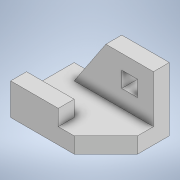
# Autodesk Inventor part: 零件12
Saved by Autodesk Inventor 2020 (Build 240168000, 168)
## iProperties
Created: 2020-09-19
Part Number: 零件12
Material: 一般
Document SubType Name: Modeling
Designer: User
Density: 1 g/cm^3
Appearance: 預設
Author: User
Autodesk Inventor part; units mm, degrees
ref_plane "YZ Plane" through (0, 0, 0) normal (1, 0, 0) x (0, 1, 0)
ref_plane "XZ Plane" through (0, 0, 0) normal (0, 1, 0) x (-1, 0, 0)
ref_plane "XY Plane" through (0, 0, 0) normal (0, 0, 1) x (1, 0, 0)
sketch "草圖1" plane through (0, 0, 0) normal (0, 0, 1) x (1, 0, 0)
  line L0 (0, 0) -> (60, 0)
  line L1 (60, 0) -> (60, 10)
  line L2 (60, 10) -> (0, 10)
  line L3 (0, 10) -> (0, 0)
  line L4 (60, 10) -> (30, 10)
  line L5 (30, 10) -> (30, 40)
  line L6 (30, 40) -> (60, 40)
  line L7 (60, 40) -> (60, 10)
  line L8 (40, 30.8819) -> (50, 30.8819)
  line L9 (50, 30.8819) -> (50, 20.8819)
  line L10 (50, 20.8819) -> (40, 20.8819)
  line L11 (40, 20.8819) -> (40, 30.8819)
  line L12 (30, 10) -> (10, 10)
  line L13 (10, 10) -> (30, 40)
  dimension "d0" = 60
  dimension "d1" = 10
  dimension "d2" = 30
  dimension "d3" = 30
  dimension "d4" = 10
  dimension "d5" = 10
  dimension "d6" = 10
  dimension "d7" = 20
  constraints: 28 end point, 6 parallel, 3 horizontal, 3 perpendicular, 1 point on line
  measures "d0" distance of L2.end L1.end
  measures "d1" distance of L1.end L0.end
  measures "d2" distance of L5.end L6.end
  measures "d3" distance of L4.end L5.end
  measures "d4" distance of L8.start L8.end
  measures "d5" distance of L10.end L8.start
  measures "d6" distance between parallel lines of L7 L9
  measures "d7" distance of L4.end L12.end
extrude "擠出1" add sketch "草圖1" along normal blind 40 contours L3 L2 L1 L0
extrude "擠出2" add sketch "草圖1" along normal blind 10 contours L2 L5 L6 L7 | L13 L5 L2
sketch "草圖2" plane through (0, 0, 40) normal (0, 0, 1) x (1, 0, 0)
  line L0 (10, 10) -> (0, 10) projected
  line L1 (0, 10) -> (30, 10)
  line L2 (30, 10) -> (30, 20)
  line L3 (30, 20) -> (0, 20)
  line L4 (0, 20) -> (0, 10)
  point P0 (0, 0)
  dimension "d12" = 30
  dimension "d13" = 10
  constraints: 8 end point, 2 parallel, 1 horizontal, 1 perpendicular
  measures "d12" distance of L3.end L2.end
  measures "d13" distance of L2.end L1.end
extrude "擠出3" add sketch "草圖2" against normal blind 10
chamfer "倒角1" distance 20 angle 45 1 edges at (60, 5, 40)
